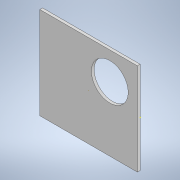
# Autodesk Inventor part: box top
Saved by Autodesk Inventor 2020 (Build 240168000, 168)
## iProperties
Created: 2020-12-15
Part Number: box top
Material: Generic
Document SubType Name: Modeling
Designer: moham
Density: 1 g/cm^3
Appearance: Default
Author: moham
Autodesk Inventor part; units mm, degrees
ref_plane "YZ Plane" through (0, 0, 0) normal (1, 0, 0) x (0, 1, 0)
ref_plane "XZ Plane" through (0, 0, 0) normal (0, 1, 0) x (-1, 0, 0)
ref_plane "XY Plane" through (0, 0, 0) normal (0, 0, 1) x (1, 0, 0)
sketch "Sketch1" plane through (0, 0, 0) normal (0, 0, 1) x (1, 0, 0)
  line L0 (-53, 50) -> (53, 50)
  line L1 (-53, 50) -> (-53, -50)
  line L2 (-53, -50) -> (53, -50)
  line L3 (53, -50) -> (53, 50)
  line L4 (0, 0) -> (-53, 0)
  line L5 (0, 0) -> (0, 50)
  line L6 (53, 50) -> (23, 50)
  line L7 (23, 50) -> (23, 20)
  circle A0 centre (23, 20) radius 20
  dimension "d0" = 106
  dimension "d1" = 100
  dimension "d2" = 53
  dimension "d12" = 50
  dimension "d13" = 30
  dimension "d14" = 30
  dimension "d15" = 40
  constraints: 16 end point, 4 perpendicular, 2 midpoint, 1 centre point, 1 coincident, 1 horizontal, 1 point on line, 1 vertical
  measures "d0" distance of L0.start L0.end
  measures "d1" distance of L0.start L1.end
  measures "d2" distance from line of L1 L4.start
  measures "d12" distance of L4.start L5.end
  measures "d13" distance of L0.end L6.end
  measures "d14" distance of L6.end L7.end
  measures "d15" diameter of A0
sketch "Sketch2" plane through (0, 0, 0) normal (0, 0, 1) x (1, 0, 0)
  point P0 (0, 0)
extrude "Extrusion1" add sketch "Sketch1" along normal blind 3 contours L0 L5 L4 L1 | L0 L3 L2 L1 L4 L5 | A0
sketch "Sketch3" plane through (53, -50, 0) normal (1, 0, 0) x (0, 0, -1)
  point P0 (0, 50)
sketch "Sketch4" plane through (0, 0, 0) normal (0, 0, 1) x (1, 0, 0)
  point P0 (0, 0)
extrude "Extrusion2" cut sketch "Sketch1" along normal through all contours A0
body "Solid1"
